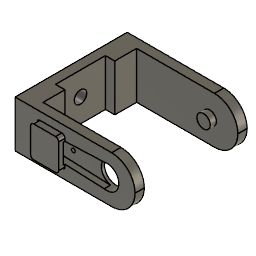
Connector_v10 (Autodesk Fusion 360 design; units mm, degrees)
Autodesk Fusion 360 part; units mm, degrees
other "기준 메쉬 피쳐2"
sketch "스케치1" plane through (0, 0, 0) normal (0, 0, 1) x (1, 0, 0)
  line L0 (-15, 36) -> (0, 36)
  line L1 (0, 36) -> (0, 0)
  line L2 (0, 0) -> (-15, 0)
  line L3 (-15, 0) -> (-15, 36)
  circle A0 centre (-7.5, 18) radius 2
  line L4 (-15, 3) -> (0, 3)
  line L5 (-15, 33) -> (0, 33)
  line L6 (-15, 26) -> (0, 26)
  line L7 (-15, 10) -> (0, 10)
  dimension "d1" = 15
  dimension "d2" = 36
  dimension "d3" = 2
  dimension "d4" = 7.5
  dimension "d5" = 18
  dimension "d6" = 3
  dimension "d7" = 3
  dimension "d8" = 10
  dimension "d9" = 10
  constraint horizontal L0
  constraint vertical L1
  constraint horizontal L2
  constraint vertical L3
  constraint coincident L1.end L2.start
  constraint coincident L3 L4.start
  constraint coincident L1 L4.end
  constraint perpendicular L1 L4
  constraint coincident L3 L5.start
  constraint coincident L1 L5.end
  constraint perpendicular L1 L5
  constraint coincident L1 L6.end
  constraint perpendicular L1 L6
  constraint coincident L3 L7.start
  constraint coincident L1 L7.end
  constraint perpendicular L1 L7
  constraint coincident L3 L6.start
  measures "d1" distance of L0.start L0.end
  measures "d2" distance of L0.start L2.end
  measures "d3" radius of A0
  measures "d4" horizontal distance of L1.end A0.centre
  measures "d5" distance of L2 A0.centre
  measures "d6" distance of L0.end L5.end
  measures "d7" distance of L1.end L4.end
  measures "d8" distance of L1.end L7.end
  measures "d9" distance of L0.end L6.end
extrude "돌출1" add sketch "스케치1" along normal blind 6 contours L1 L3 L5 L6 | L1 L3 L4 L7 makes body 1 at (-10, 7.6667, 0) makes body 2 at (-10, 30.6667, 0)
extrude "돌출2" add sketch "스케치1" along normal blind 38.5 contours L0 L1 L3 L5 | L1 L2 L3 L4 bodies 1 2
extrude "돌출3" add sketch "스케치1" along normal blind 3 contours L1 L3 L6 L7 bodies 1 2
sketch "스케치3" plane through (0, 0, 0) normal (0, -1, 0) x (1, 0, 0)
  line L0 (0, 0) -> (-15, 0)
  arc A0 (-10.5974, 13.8736) -> (-4.4026, 13.8736) centre (-7.5, 14) ccw
  circle A1 centre (-7.5, 16.7) radius 0.6
  line L1 (-15, 6) -> (-15, 38.5)
  line L2 (0, 6) -> (0, 38.5)
  line L3 (-15, 16) -> (0, 16)
  line L4 (-12.5, 16) -> (-12.5, 7)
  line L5 (-12.5, 7) -> (-2.5, 7)
  line L6 (-2.5, 7) -> (-2.5, 16)
  circle A2 centre (-7.5, 29.5) radius 3.8
  line L7 (-10.5974, 13.8736) -> (-11.2, 28.634)
  line L8 (-4.4026, 13.8736) -> (-3.8, 28.634)
  line L9 (0, 38.5) -> (-15, 38.5)
  point P0 (-7.5, 0)
  point P1 (-7.5, 7)
  point P2 (-7.5, 0)
  dimension "d24" = 6.2
  dimension "d26" = 15.5
  dimension "d28" = 1.2
  dimension "d29" = 12.8
  dimension "d30" = 16
  dimension "d33" = 9
  dimension "d34" = 10
  dimension "d35" = 14
  dimension "d36" = 7.6
  dimension "d37" = 7.4
  constraint midpoint L0 P2
  constraint coincident L1 L3.start
  constraint coincident L2 L3.end
  constraint coincident L3 L4.start
  constraint perpendicular L3 L4
  constraint perpendicular L4 L5
  constraint coincident L3 L6.end
  constraint perpendicular L3 L6
  constraint midpoint L5 P1
  constraint horizontal L3
  constraint coincident A2 L7.end
  constraint coincident A2 L8.end
  constraint horizontal L7.end L8.end
  constraint vertical A0.centre A2.centre
  constraint vertical P1 A2.centre
  constraint vertical A2.centre P2
  constraint tangent A0 L8
  constraint tangent A0 L7
  constraint vertical A1.centre A2.centre
  measures "d24" diameter of A0
  measures "d26" distance of A0.centre A2.centre
  measures "d28" diameter of A1
  measures "d29" vertical distance of A1.centre A2.centre
  measures "d30" distance of L0.start L3.end
  measures "d33" distance of L4.start L4.end
  measures "d34" distance of L4.end L5.end
  measures "d35" distance of P2 A0.centre
  measures "d36" diameter of A2
  measures "d37" distance of L7.end L8.end
extrude "돌출5" cut sketch "스케치3" against normal blind 3 contours A2 bodies 1
extrude "돌출6" cut sketch "스케치3" against normal blind 3 contours A1 bodies 1
extrude "돌출7" cut sketch "스케치3" against normal blind 2 contours A0 L3 L7 L8 | L3 A2 L7 L8 bodies 1
extrude "돌출8" add sketch "스케치3" along normal blind 2 contours A0 L3 L7 L8 | A0 L3 L4 L5 L6 L7 L8 bodies 1
extrude "돌출9" cut sketch "스케치3" along normal blind 0.5 contours A0 L3 L7 L8 bodies 1
fillet "필렛1" radius 1 4 edges at (-2.5, -1, 7) (-2.5, -1, 16) (-12.5, -1, 16) (-12.5, -1, 7) on bodies 1
fillet "필렛3" radius 7.5 2 edges at (0, 1.5, 38.5) (-15, 1.5, 38.5) on bodies 1
sketch "스케치9" plane through (0, 33, 0) normal (0, -1, 0) x (1, 0, 0)
  arc A0 (0, 31) -> (-7.5, 38.5) centre (-7.5, 31) ccw
  arc A1 (-7.5, 38.5) -> (-15, 31) centre (-7.5, 31) ccw
  arc A2 (-3.8, 28.634) -> (-11.2, 28.634) centre (-7.5, 29.5) ccw
  circle A3 centre (-7.5, 29.5) radius 2.15
  dimension "d55" = 4.3
  constraint concentric A2 A3
  measures "d55" diameter of A3
extrude "돌출10" add sketch "스케치9" along normal blind 2 bodies 1
fillet "필렛4" radius 7.5 2 edges at (0, 34.5, 38.5) (-15, 34.5, 38.5) on bodies 1
move_body "이동1" bodies 1 to x (0, 0, -1) y (0, 1, 0) z (1, 0, 0) at (-6, 0, 6)
